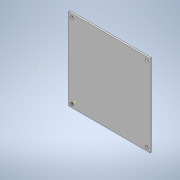
# Autodesk Inventor part: bottomplate
Saved by Autodesk Inventor 2022 (Build 260153000, 153)
## iProperties
Created: 2023-12-05
Part Number: bottomplate
Material: Generisch
Document SubType Name: Modeling
Designer: Marc Panse
Density: 1 g/cm^3
Appearance: Vorgabe
Author: Marc Panse
## iProperties of the stored document bottomplate_3D-Druck.ipt
Created: 2023-12-05
Part Number: bottomplate_3D-Druck
Material: Generisch
Document SubType Name: Modeling
Designer: Marc Panse
Density: 1 g/cm^3
Appearance: Vorgabe
Author: Marc Panse
Autodesk Inventor part; units mm, degrees
ref_plane "YZ Plane" through (0, 0, 0) normal (1, 0, 0) x (0, 1, 0)
ref_plane "XZ Plane" through (0, 0, 0) normal (0, 1, 0) x (-1, 0, 0)
ref_plane "XY Plane" through (0, 0, 0) normal (0, 0, 1) x (1, 0, 0)
sketch "Skizze1" plane through (0, 0, 0) normal (0, 0, 1) x (1, 0, 0)
  line L0 (-33.02, -33.02) -> (33.02, -33.02)
  line L1 (33.02, -33.02) -> (33.02, 33.02)
  line L2 (33.02, 33.02) -> (-33.02, 33.02)
  line L3 (-33.02, 33.02) -> (-33.02, -33.02)
  line L4 (-33.02, -33.02) -> (33.02, 33.02) construction
  line L5 (33.02, -33.02) -> (-33.02, 33.02) construction
  line L6 (-34, -34) -> (34, -34)
  line L7 (34, -34) -> (34, 34)
  line L8 (34, 34) -> (-34, 34)
  line L9 (-34, 34) -> (-34, -34)
  line L10 (-34, -34) -> (34, 34) construction
  line L11 (34, -34) -> (-34, 34) construction
  point P0 (0, 0)
  dimension "d0" = 66.04
  dimension "d1" = 66.04
  dimension "d2" = 68
  dimension "d3" = 68
  constraints: 24 end point, 4 midpoint, 4 parallel, 2 horizontal, 2 perpendicular
  measures "d0" distance of L2.end L1.end
  measures "d1" distance of L1.end L0.end
  measures "d2" distance of L8.end L7.end
  measures "d3" distance of L7.end L6.end
extrude "Extrusion1" add sketch "Skizze1" along normal blind 6.5
sketch "Skizze2" plane through (0, 0, 6.5) normal (0, 0, 1) x (1, 0, 0)
  line L0 (-33.02, 33.02) -> (33.02, 33.02) projected
  line L1 (-33.02, -33.02) -> (33.02, -33.02)
  line L2 (33.02, -33.02) -> (33.02, 33.02)
  line L3 (33.02, 33.02) -> (-33.02, 33.02)
  line L4 (-33.02, 33.02) -> (-33.02, -33.02)
  line L5 (-33.02, -33.02) -> (33.02, 33.02) construction
  line L6 (33.02, -33.02) -> (-33.02, 33.02) construction
  line L7 (34, -34) -> (34, 34) projected
  line L8 (34, 34) -> (-34, 34) projected
  line L9 (-34, 34) -> (-34, -34) projected
  line L10 (-34, -34) -> (34, -34) projected
  line L11 (-33.02, -33.02) -> (-33.02, 33.02) projected
  line L12 (-33.02, 33.02) -> (33.02, 33.02) projected
  line L13 (33.02, 33.02) -> (33.02, -33.02) projected
  line L14 (33.02, -33.02) -> (-33.02, -33.02) projected
  point P0 (0, 0)
  constraints: 12 end point, 2 midpoint, 2 parallel, 1 horizontal, 1 perpendicular
extrude "Extrusion2" add sketch "Skizze2" along normal blind 2 contours L0 L2 L1 L4 | L10 L9 L8 L7
sketch "Skizze3" plane through (0, 0, 6.5) normal (0, 0, -1) x (-1, 0, 0)
  line L0 (-27.94, -27.94) -> (27.94, -27.94)
  line L1 (27.94, -27.94) -> (27.94, 27.94)
  line L2 (27.94, 27.94) -> (-27.94, 27.94)
  line L3 (-27.94, 27.94) -> (-27.94, -27.94)
  line L4 (-27.94, -27.94) -> (27.94, 27.94) construction
  line L5 (27.94, -27.94) -> (-27.94, 27.94) construction
  circle A0 centre (-27.94, 27.94) radius 3.35
  circle A1 centre (27.94, 27.94) radius 3.35
  circle A2 centre (27.94, -27.94) radius 3.35
  circle A3 centre (-27.94, -27.94) radius 3.35
  point P0 (0, 0)
  dimension "d8" = 55.88
  dimension "d9" = 55.88
  dimension "d10" = 6.7
  dimension "d11" = 6.7
  dimension "d12" = 6.7
  dimension "d13" = 6.7
  constraints: 12 end point, 4 centre point, 4 coincident, 2 midpoint, 2 parallel, 1 horizontal, 1 perpendicular
  measures "d8" distance of L2.end L1.end
  measures "d9" distance of L1.end L0.end
  measures "d10" diameter of A0
  measures "d11" diameter of A1
  measures "d12" diameter of A2
  measures "d13" diameter of A3
extrude "Extrusion3" add sketch "Skizze3" along normal blind 5 contours L3 A3 L0 | L0 A3 L3 | A2 L1 L0 | L0 L1 A2 | A0 L2 L3 | L3 L2 A0 | A1 L2 L1 | L1 L2 A1
sketch "Skizze4" plane through (27.94, 27.94, 1.5) normal (0, 0, -1) x (-1, 0, 0)
  circle A0 centre (0, 0) radius 1.1
  circle A1 centre (55.88, 0) radius 3.35 projected
  circle A2 centre (55.88, 0) radius 1.1
  circle A3 centre (55.88, -55.88) radius 3.35 projected
  circle A4 centre (55.88, -55.88) radius 1.1
  circle A5 centre (0, -55.88) radius 3.35 projected
  circle A6 centre (0, -55.88) radius 1.1
  point P0 (27.94, -27.94)
  dimension "d17" = 2.2
  dimension "d18" = 2.2
  dimension "d19" = 2.2
  dimension "d20" = 2.2
  constraints: 4 centre point, 3 coincident
  measures "d17" diameter of A0
  measures "d18" diameter of A2
  measures "d19" diameter of A4
  measures "d20" diameter of A6
extrude "Extrusion4" cut sketch "Skizze4" against normal blind 5 contours A0 | A2 | A4 | A6
sketch "Skizze5" plane through (0, 0, 0) normal (0, 0, -1) x (-1, 0, 0)
  line L0 (-34, -34) -> (-34, 34) projected
  line L1 (34, -34) -> (-34, -34) projected
  line L2 (34, 34) -> (34, -34) projected
  line L3 (-34, 34) -> (34, 34) projected
  line L4 (33.02, -33.02) -> (33.02, 33.02) projected
  line L5 (-33.02, -33.02) -> (33.02, -33.02) projected
  line L6 (-33.02, 33.02) -> (-33.02, -33.02) projected
  line L7 (33.02, 33.02) -> (-33.02, 33.02) projected
  point P0 (0, 0)
extrude "Extrusion5" add sketch "Skizze5" along normal blind 4
sketch "Skizze6" plane through (0, 0, -4) normal (0, 0, -1) x (-1, 0, 0)
  line L0 (-33.02, -33.02) -> (33.02, -33.02)
  line L1 (33.02, -33.02) -> (33.02, 33.02)
  line L2 (33.02, 33.02) -> (-33.02, 33.02)
  line L3 (-33.02, 33.02) -> (-33.02, -33.02)
  line L4 (-33.02, -33.02) -> (33.02, 33.02) construction
  line L5 (33.02, -33.02) -> (-33.02, 33.02) construction
  line L6 (33.02, -33.02) -> (20.02, -33.02)
  line L7 (-33.02, -33.02) -> (33.02, -33.02) projected
  line L8 (20.02, -33.02) -> (10.08, -33.02)
  line L9 (34, -34) -> (-34, -34) projected
  line L10 (10.08, -33.02) -> (20.02, -33.02)
  line L11 (20.02, -33.02) -> (20.02, -34)
  line L12 (20.02, -34) -> (10.08, -34)
  line L13 (10.08, -34) -> (10.08, -33.02)
  point P0 (0, 0)
  point P1 (-24.13, -33.02)
  point P2 (24.13, -33.02)
  dimension "d25" = 66.04
  dimension "d26" = 66.04
  dimension "d27" = 13
  dimension "d28" = 9.94
  constraints: 24 end point, 4 parallel, 3 point on line, 2 horizontal, 2 midpoint, 2 perpendicular
  measures "d25" distance of L2.end L1.end
  measures "d26" distance of L1.end L0.end
  measures "d27" distance of L0.end L6.end
  measures "d28" distance of L6.end L8.end
extrude "Extrusion6" cut sketch "Skizze6" against normal blind 4 contours L0 L11 L9 L13
fillet "Rundung2" radius 1.75 2 edges at (-10.08, -33.51, 0) (-20.02, -33.51, 0)
sketch "Skizze7" plane through (0, 0, -4) normal (0, 0, -1) x (-1, 0, 0)
  line L0 (34, 34) -> (-34, 34) projected
  line L1 (-34, -34) -> (34, -34)
  line L2 (34, -34) -> (34, 34)
  line L3 (34, 34) -> (-34, 34)
  line L4 (-34, 34) -> (-34, -34)
  line L5 (-34, -34) -> (34, 34) construction
  line L6 (34, -34) -> (-34, 34) construction
  line L7 (-35, -35) -> (35, -35)
  line L8 (35, -35) -> (35, 35)
  line L9 (35, 35) -> (-35, 35)
  line L10 (-35, 35) -> (-35, -35)
  line L11 (-35, -35) -> (35, 35) construction
  line L12 (35, -35) -> (-35, 35) construction
  point P0 (0, 0)
  point P1 (-34, 34)
  dimension "d32" = 70
  dimension "d33" = 70
  constraints: 24 end point, 4 midpoint, 4 parallel, 2 horizontal, 2 perpendicular
  measures "d32" distance of L9.end L8.end
  measures "d33" distance of L8.end L7.end
extrude "Extrusion7" add sketch "Skizze7" against normal up to surface (12.5 mm away)
sketch "Skizze8" plane through (-20.02, -34, -4) normal (0, 1, 0) x (1, 0, 0)
  line L0 (9.94, -2.25) -> (9.94, 0) projected
  line L1 (0, 0) -> (9.94, 0) projected
  line L2 (0, 0) -> (0, -2.25) projected
  arc A0 (0, -2.25) -> (1.75, -4) centre (1.75, -2.25) ccw projected
  line L3 (1.75, -4) -> (8.19, -4) projected
  arc A1 (8.19, -4) -> (9.94, -2.25) centre (8.19, -2.25) ccw projected
  point P0 (20.02, -4)
extrude "Extrusion8" cut sketch "Skizze8" against normal blind 10
sketch "Skizze9" plane through (0, 0, -4) normal (0, 0, -1) x (-1, 0, 0)
  line L0 (-33.52, 33.52) -> (33.52, 33.52)
  line L1 (33.52, 33.52) -> (33.52, -33.52)
  line L2 (33.52, -33.52) -> (-33.52, -33.52)
  line L3 (-33.52, -33.52) -> (-33.52, 33.52)
  line L4 (-33.52, 33.52) -> (33.52, -33.52) construction
  line L5 (33.52, 33.52) -> (-33.52, -33.52) construction
  line L6 (10.08, -35) -> (10.08, -33.02) projected
  line L7 (10.08, -33.02) -> (-33.02, -33.02) projected
  line L8 (-33.02, -33.02) -> (-33.02, 33.02) projected
  line L9 (-33.02, 33.02) -> (33.02, 33.02) projected
  line L10 (33.02, 33.02) -> (33.02, -33.02) projected
  line L11 (33.02, -33.02) -> (20.02, -33.02) projected
  line L12 (20.02, -33.02) -> (20.02, -35) projected
  line L13 (20.02, -35) -> (35, -35) projected
  line L14 (35, -35) -> (35, 35) projected
  line L15 (35, 35) -> (-35, 35) projected
  line L16 (-35, 35) -> (-35, -35) projected
  line L17 (-35, -35) -> (10.08, -35) projected
  point P0 (0, 0)
  point P1 (10.08, -33.52)
  point P2 (20.02, -33.52)
  dimension "d38" = 67.04
  dimension "d39" = 67.04
  constraints: 12 end point, 2 midpoint, 2 parallel, 1 horizontal, 1 perpendicular
  measures "d38" distance of L1.end L2.end
  measures "d39" distance of L0.end L1.end
extrude "Extrusion9" cut sketch "Skizze9" against normal up to surface (10.5 mm away) contours L0 L1 L2 L12 L11 L10 L9 L8 L7 L6 L3
fillet "Rundung3" radius 2 4 edges at (31.29, -27.94, 6.5) (31.29, 27.94, 6.5) (-24.59, 27.94, 6.5) (-24.59, -27.94, 6.5)
sketch "Skizze10" plane through (-35, -35, -4) normal (-1, 0, 0) x (0, 0, 1)
  point P0 (4, 35)
sketch "Skizze11" plane through (0, 0, 8.5) normal (0, 0, 1) x (1, 0, 0)
  point P0 (0, 0)
sketch "Skizze12" plane through (-18.27, -33.02, 0) normal (0, 1, 0) x (1, 0, 0)
  line L0 (-1.75, 1.75) -> (-1.75, -6.5) projected
  line L1 (8.19, -6.5) -> (-1.75, -6.5) projected
  line L2 (8.19, -6.5) -> (8.19, 1.75) projected
  arc A0 (6.44, 0) -> (8.19, 1.75) centre (6.44, 1.75) ccw projected
  line L3 (6.44, 0) -> (0, 0) projected
  arc A1 (-1.75, 1.75) -> (0, 0) centre (0, 1.75) ccw projected
  point P0 (18.27, 0)
extrude "Extrusion10" cut sketch "Skizze12" against normal up to surface (0.5 mm away)
sketch "Skizze13" plane through (0, 0, -4) normal (0, 0, -1) x (-1, 0, 0)
  circle A0 centre (0, 0) radius 4
  line L0 (0, 0) -> (-10.0581, 1.7135)
  line L1 (0, 0) -> (10.203, 0) construction
  line L2 (0, 0) -> (1.8539, 9.7483)
  line L3 (0, 0) -> (9.923, 0) construction
  line L4 (0, 0) -> (9.888, -2.1637)
  line L5 (0, 0) -> (10.122, 0) construction
  line L6 (0, 0) -> (-2.0234, -10.1982)
  line L7 (0, 0) -> (10.397, 0) construction
  circle A1 centre (-2.0234, -10.1982) radius 2.5
  circle A2 centre (-10.0581, 1.7135) radius 2.5
  circle A3 centre (1.8539, 9.7483) radius 2.5
  circle A4 centre (9.888, -2.1637) radius 2.5
  dimension "d59" = 8
  dimension "d60" = 10.203
  dimension "d61" = 170.332
  dimension "d62" = 9.923
  dimension "d63" = 79.232
  dimension "d64" = 10.122
  dimension "d65" = 12.343
  dimension "d66" = 10.397
  dimension "d67" = 101.222
  dimension "d68" = 5
  dimension "d69" = 5
  dimension "d70" = 5
  dimension "d71" = 5
  constraints: 16 end point, 5 centre point, 5 coincident, 4 equal length, 4 horizontal
  measures "d59" diameter of A0
  measures "d60" distance of L0.start L0.end
  measures "d61" angle of L1 L0
  measures "d62" distance of L0.start L2.end
  measures "d63" angle of L3 L2
  measures "d64" distance of L0.start L4.end
  measures "d65" angle of L4 L5
  measures "d66" distance of L0.start L6.end
  measures "d67" angle of L6 L7
  measures "d68" diameter of A1
  measures "d69" diameter of A2
  measures "d70" diameter of A3
  measures "d71" diameter of A4
extrude "Extrusion11" add sketch "Skizze13" against normal up to surface (10.5 mm away) contours A1 | A2 | A3 | A4
sketch "Skizze14" plane through (-9.888, -2.1637, -4) normal (0, 0, -1) x (-1, 0, 0)
  circle A0 centre (0, 0) radius 2.5 projected
  circle A1 centre (-11.9114, -8.0345) radius 2.5 projected
  circle A2 centre (-19.9461, 3.8772) radius 2.5 projected
  circle A3 centre (-8.0341, 11.912) radius 2.5 projected
  point P0 (-9.888, 2.1637)
extrude "Extrusion12" cut sketch "Skizze14" against normal blind 5.5
fillet "Rundung4" radius 4 4 edges at (12.5581, 1.7135, 6.5) (0.6461, 9.7483, 6.5) (-7.388, -2.1637, 6.5) (4.5234, -10.1982, 6.5)
sketch "Skizze15" plane through (-9.888, -2.1637, 1.5) normal (0, 0, -1) x (-1, 0, 0)
  circle A0 centre (0, 0) radius 1
  circle A1 centre (-11.9114, -8.0345) radius 2.5 projected
  circle A2 centre (-11.9114, -8.0345) radius 1
  circle A3 centre (-19.9461, 3.8772) radius 2.5 projected
  circle A4 centre (-19.9461, 3.8772) radius 1
  circle A5 centre (-8.0341, 11.912) radius 2.5 projected
  circle A6 centre (-8.0341, 11.912) radius 1
  point P0 (-9.888, 2.1637)
  dimension "d77" = 2
  dimension "d78" = 2
  dimension "d79" = 2
  dimension "d80" = 2
  constraints: 4 centre point, 3 coincident
  measures "d77" diameter of A0
  measures "d78" diameter of A2
  measures "d79" diameter of A4
  measures "d80" diameter of A6
extrude "Extrusion13" cut sketch "Skizze15" against normal blind 5 contours A0 | A2 | A4 | A6
chamfer "Fase1" distance 4 angle 45 4 edges at (-33.52, 0, 6.5) (0, -33.52, 6.5) (0, 33.52, 6.5) (33.52, 0, 6.5)
sketch "Skizze16" plane through (10.0581, 1.7135, 1.5) normal (0, 0, -1) x (-1, 0, 0)
  circle A0 centre (0, 0) radius 1.6
  circle A1 centre (8.0347, -11.9117) radius 1 projected
  circle A2 centre (8.0347, -11.9117) radius 1.6
  circle A3 centre (11.912, 8.0348) radius 1 projected
  circle A4 centre (11.912, 8.0348) radius 1.6
  circle A5 centre (19.9461, -3.8772) radius 1 projected
  circle A6 centre (19.9461, -3.8772) radius 1.6
  point P0 (10.0581, -1.7135)
  dimension "d86" = 3.2
  dimension "d87" = 3.2
  dimension "d88" = 3.2
  dimension "d89" = 3.2
  constraints: 4 centre point, 3 coincident
  measures "d86" diameter of A0
  measures "d87" diameter of A2
  measures "d88" diameter of A4
  measures "d89" diameter of A6
extrude "Extrusion14" cut sketch "Skizze16" against normal blind 10 contours A0 | A1 | A2 | A3 | A4 | A5 | A6
chamfer "Fase2" distance 2 angle 45 4 edges at (-8.288, -2.1637, 8.5) (3.6234, -10.1982, 8.5) (11.6581, 1.7135, 8.5) (-0.2539, 9.7483, 8.5)
sketch "Skizze17" plane through (27.94, 27.94, 1.5) normal (0, 0, -1) x (-1, 0, 0)
  circle A0 centre (0, 0) radius 1.1 projected
  circle A1 centre (0, 0) radius 3.35 projected
  circle A2 centre (55.88, 0) radius 1.1 projected
  circle A3 centre (55.88, 0) radius 3.35 projected
  circle A4 centre (55.88, -55.88) radius 1.1 projected
  circle A5 centre (55.88, -55.88) radius 3.35 projected
  circle A6 centre (0, -55.88) radius 1.1 projected
  circle A7 centre (0, -55.88) radius 3.35 projected
  line L0 (61.46, 5.58) -> (58.4446, 2.5646) projected
  line L1 (-2.5646, -58.4446) -> (58.4446, -58.4446)
  line L2 (58.4446, -58.4446) -> (58.4446, 2.5646)
  line L3 (58.4446, 2.5646) -> (-2.5646, 2.5646)
  line L4 (-2.5646, 2.5646) -> (-2.5646, -58.4446)
  line L5 (-2.5646, -58.4446) -> (58.4446, 2.5646) construction
  line L6 (58.4446, -58.4446) -> (-2.5646, 2.5646) construction
  point P0 (27.94, -27.94)
  constraints: 12 end point, 2 midpoint, 2 parallel, 1 horizontal, 1 perpendicular
extrude "Extrusion15" add sketch "Skizze17" along normal blind 20 contours A1 L4 L3 | A1 L3 A3 L2 A5 L1 A7 L4 | A1 L4 L3 | L3 A3 L2 | A7 L1 L4 | L3 L2 A3 | A7 L1 L4 | L2 A5 L1 | L2 L1 A5
sketch "Skizze18" plane through (0, 0, 8.5) normal (0, 0, 1) x (1, 0, 0)
  line L0 (-192.7529, 161.1187) -> (54.5088, 161.1187)
  line L1 (54.5088, 161.1187) -> (54.5088, -50.2743)
  line L2 (54.5088, -50.2743) -> (-192.7529, -50.2743)
  line L3 (-192.7529, -50.2743) -> (-192.7529, 161.1187)
  line L4 (-192.7529, 161.1187) -> (54.5088, -50.2743) construction
  line L5 (54.5088, 161.1187) -> (-192.7529, -50.2743) construction
  point P0 (0, 0)
  point P1 (-69.122, 55.4222)
  constraints: 12 end point, 2 midpoint, 2 parallel, 1 horizontal, 1 perpendicular
extrude "Extrusion16" cut sketch "Skizze18" against normal blind 25.75
